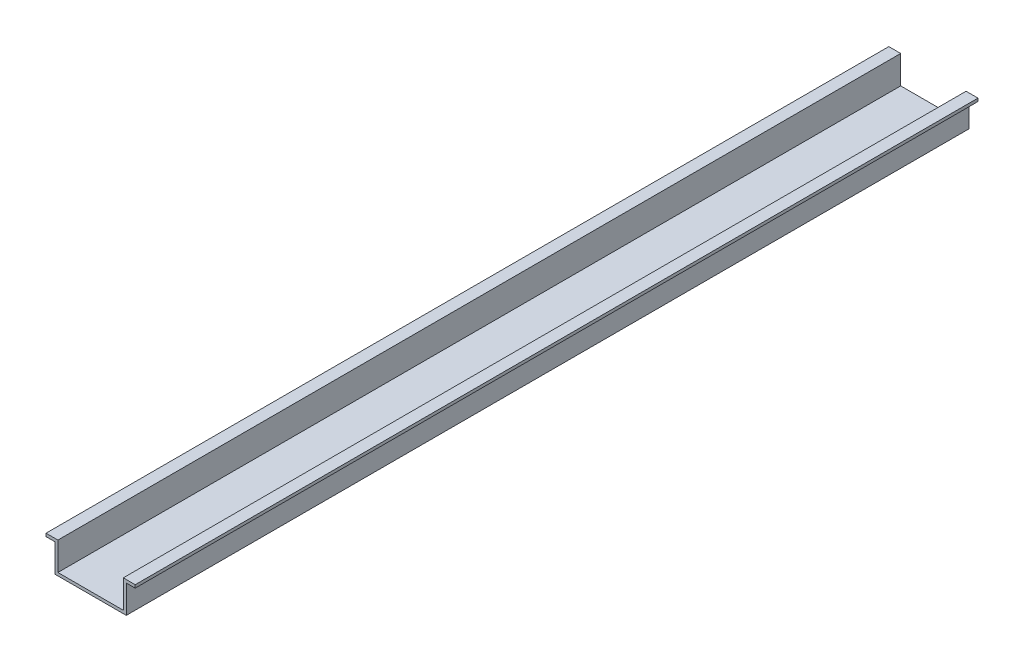
# Autodesk Inventor part: C_CHANNEL
Saved by Autodesk Inventor 2023 (Build 270158000, 158)
## iProperties
Created: 2024-08-24
Part Number: C_CHANNEL
Material: Generic
Document SubType Name: Modeling
Designer: think
Density: 1 g/cm^3
Appearance: Default
Author: think
Autodesk Inventor part; units mm, degrees
ref_plane "YZ Plane" through (0, 0, 0) normal (1, 0, 0) x (0, 1, 0)
ref_plane "XZ Plane" through (0, 0, 0) normal (0, 1, 0) x (-1, 0, 0)
ref_plane "XY Plane" through (0, 0, 0) normal (0, 0, 1) x (1, 0, 0)
sketch "Sketch1" plane through (0, 0, 0) normal (0, 0, 1) x (1, 0, 0)
  line L0 (0, 0) -> (0, 30)
  line L1 (0, 30) -> (-9.525, 30)
  line L2 (-9.525, 30) -> (-9.525, 33.175)
  line L3 (-9.525, 33.175) -> (3.175, 33.175)
  line L4 (3.175, 33.175) -> (3.175, 3.175)
  line L5 (3.175, 3.175) -> (73.025, 3.175)
  line L6 (73.025, 3.175) -> (73.025, 33.175)
  line L7 (73.025, 33.175) -> (85.725, 33.175)
  line L8 (85.725, 33.175) -> (85.725, 30)
  line L9 (85.725, 30) -> (76.2, 30)
  line L10 (76.2, 30) -> (76.2, 0)
  line L11 (76.2, 0) -> (0, 0)
  dimension "d0" = 76.2
  dimension "d1" = 3.175
  dimension "d2" = 3.175
  dimension "d3" = 3.175
  dimension "d5" = 30
  dimension "d8" = 12.7
  constraints: 24 end point, 10 perpendicular, 3 equal length, 2 point on line, 1 vertical
  measures "d0" distance of L10.end L0.start
  measures "d1" distance between parallel lines of L11 L5
  measures "d2" distance between parallel lines of L10 L6
  measures "d3" distance of L7.end L8.end
  measures "d5" distance of L3.end L4.end
  measures "d8" distance between parallel lines of L4 L2
extrude "Extrusion1" add sketch "Sketch1" along normal blind 900
body "Solid1"
